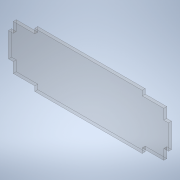
# Autodesk Inventor part: 103.011.01_Abdeckung_Gestell_seitlich
Saved by Autodesk Inventor 2021 (Build 250183000, 183)
## iProperties
Created: 2021-11-25
Part Number: 103.011.01_Abdeckung_Gestell_seitlich
Material: PMMA-Kunststoff
Document SubType Name: Modeling
Designer: Sebastian Seewald
Mass: 65.5279 g
Surface Area: 298.591 cm^2
Volume: 55.1582 cm^3
Density: 1.188 g/cm^3
Appearance: Polycarbonat - klar
Author: Sebastian Seewald
Autodesk Inventor part; units mm, degrees
ref_plane "YZ Plane" through (0, 0, 0) normal (1, 0, 0) x (0, 1, 0)
ref_plane "XZ Plane" through (0, 0, 0) normal (0, 1, 0) x (-1, 0, 0)
ref_plane "XY Plane" through (0, 0, 0) normal (0, 0, 1) x (1, 0, 0)
sketch "Skizze1" plane through (0, 0, 0) normal (0, 0, 1) x (1, 0, 0)
  line L0 (0, 0) -> (212.5, 0)
  line L1 (212.5, 0) -> (212.5, 72.5)
  line L2 (212.5, 72.5) -> (0, 72.5)
  line L3 (0, 72.5) -> (0, 0)
  line L4 (0, 72.5) -> (35, 72.5)
  line L5 (35, 72.5) -> (35, 66.15)
  line L6 (35, 66.15) -> (0, 66.15)
  line L7 (0, 66.15) -> (0, 72.5)
  line L8 (0, 72.5) -> (6.35, 72.5)
  line L9 (6.35, 72.5) -> (6.35, 52.5)
  line L10 (6.35, 52.5) -> (0, 52.5)
  line L11 (0, 52.5) -> (0, 72.5)
  line L12 (0, 36.25) -> (212.5, 36.25) construction
  line L13 (106.25, 72.5) -> (106.25, 0) construction
  line L14 (0, 0) -> (35, 0)
  line L15 (35, 0) -> (35, 6.35)
  line L16 (35, 6.35) -> (0, 6.35)
  line L17 (0, 6.35) -> (0, 0)
  line L18 (0, 0) -> (6.35, 0)
  line L19 (6.35, 0) -> (6.35, 20)
  line L20 (6.35, 20) -> (0, 20)
  line L21 (0, 20) -> (0, 0)
  line L22 (212.5, 72.5) -> (212.5, 0)
  line L23 (212.5, 72.5) -> (177.5, 72.5)
  line L24 (177.5, 72.5) -> (177.5, 66.15)
  line L25 (177.5, 66.15) -> (212.5, 66.15)
  line L26 (212.5, 66.15) -> (212.5, 72.5)
  line L27 (212.5, 72.5) -> (206.15, 72.5)
  line L28 (206.15, 72.5) -> (206.15, 52.5)
  line L29 (206.15, 52.5) -> (212.5, 52.5)
  line L30 (212.5, 52.5) -> (212.5, 72.5)
  line L31 (212.5, 0) -> (206.15, 0)
  line L32 (212.5, 0) -> (177.5, 0)
  line L33 (177.5, 0) -> (177.5, 6.35)
  line L34 (177.5, 6.35) -> (212.5, 6.35)
  line L35 (206.15, 0) -> (206.15, 20)
  line L36 (212.5, 6.35) -> (212.5, 0)
  line L37 (206.15, 20) -> (212.5, 20)
  line L38 (212.5, 20) -> (212.5, 0)
  point P0 (212.5, 52.5)
  point P1 (206.15, 66.15)
  point P2 (6.35, 66.15)
  point P3 (0, 52.5)
  point P4 (0, 20)
  point P5 (6.35, 6.35)
  point P6 (206.15, 6.35)
  dimension "d0" = 212.5
  dimension "d1" = 72.5
  dimension "d2" = 35
  dimension "d3" = 6.35
  dimension "d4" = 6.35
  dimension "d5" = 20
  constraints: 78 end point, 18 symmetric about line, 6 parallel, 4 midpoint, 3 horizontal, 3 perpendicular
  measures "d0" distance of L1.end L2.end
  measures "d1" distance between parallel lines of L0 L2
  measures "d2" distance between parallel lines of L3 L5
  measures "d3" distance between parallel lines of L2 L6
  measures "d4" distance between parallel lines of L3 L9
  measures "d5" distance between parallel lines of L2 L10
extrude "Extrusion1" add sketch "Skizze1" along normal blind 4 contours L15 L16 L19 L20 L3 L10 L9 L6 L5 L2 L24 L25 L28 L29 L1 L37 L35 L34 L33 L0
